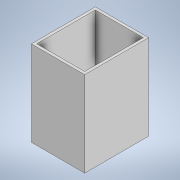
# Autodesk Inventor part: spacer
Saved by Autodesk Inventor 2022.1 (Build 261234000, 234)
## iProperties
Created: 2021-08-08
Part Number: spacer
Material: Generic
Document SubType Name: Modeling
Designer: robst
Density: 1 g/cm^3
Appearance: Default
Author: robst
Autodesk Inventor part; units mm, degrees
ref_plane "YZ Plane" through (0, 0, 0) normal (1, 0, 0) x (0, 1, 0)
ref_plane "XZ Plane" through (0, 0, 0) normal (0, 1, 0) x (-1, 0, 0)
ref_plane "XY Plane" through (0, 0, 0) normal (0, 0, 1) x (1, 0, 0)
sketch "Sketch1" plane through (0, 0, 0) normal (0, 1, 0) x (-1, 0, 0)
  line L0 (-31.75, 38.1) -> (-31.75, -38.1)
  line L1 (-31.75, -38.1) -> (31.75, -38.1)
  line L2 (31.75, -38.1) -> (31.75, 38.1)
  line L3 (31.75, 38.1) -> (-31.75, 38.1)
  line L4 (-31.75, 38.1) -> (31.75, -38.1) construction
  line L5 (-31.75, -38.1) -> (31.75, 38.1) construction
  line L6 (-28.575, 34.925) -> (-28.575, -34.925)
  line L7 (-28.575, -34.925) -> (28.575, -34.925)
  line L8 (28.575, -34.925) -> (28.575, 34.925)
  line L9 (28.575, 34.925) -> (-28.575, 34.925)
  line L10 (-28.575, 34.925) -> (28.575, -34.925) construction
  line L11 (-28.575, -34.925) -> (28.575, 34.925) construction
  point P0 (0, 0)
  dimension "d0" = 76.2
  dimension "d1" = 63.5
  dimension "d2" = 3.175
  dimension "d3" = 3.175
  constraints: 24 end point, 5 parallel, 4 midpoint, 2 perpendicular, 1 vertical
  measures "d0" distance of L1.end L2.end
  measures "d1" distance of L2.end L0.start
  measures "d2" distance between parallel lines of L2 L8
  measures "d3" distance between parallel lines of L1 L7
extrude "Extrusion1" add sketch "Sketch1" along normal blind 101.6
body "Solid1"
